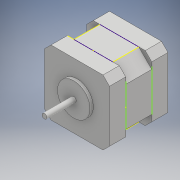
# Autodesk Inventor part: Moteur courroie
Saved by Autodesk Inventor 2018 (Build 220112000, 112)
## iProperties
Created: 2018-04-06
Part Number: Moteur courroie
Material: Générique
Document SubType Name: Modeling
Designer: Dimitri
Density: 1 g/cm^3
Appearance: Par défaut
Author: Dimitri
Autodesk Inventor part; units mm, degrees
ref_plane "YZ Plane" through (0, 0, 0) normal (1, 0, 0) x (0, 1, 0)
ref_plane "XZ Plane" through (0, 0, 0) normal (0, 1, 0) x (-1, 0, 0)
ref_plane "XY Plane" through (0, 0, 0) normal (0, 0, 1) x (1, 0, 0)
sketch "Esquisse1" plane through (0, 0, 0) normal (0, 1, 0) x (-1, 0, 0)
  line L0 (-20, 20) -> (20, 20)
  line L1 (20, 20) -> (20, -20)
  line L2 (20, -20) -> (-20, -20)
  line L3 (-20, -20) -> (-20, 20)
  line L4 (-20, 20) -> (20, -20) construction
  line L5 (20, 20) -> (-20, -20) construction
  point P0 (0, 0)
  dimension "d0" = 40
  dimension "d1" = 40
  constraints: 12 end point, 2 midpoint, 2 parallel, 1 horizontal, 1 perpendicular
  measures "d0" distance of L0.end L1.end
  measures "d1" distance of L1.end L2.end
extrude "Extrusion1" add sketch "Esquisse1" along normal blind 16
chamfer "Chanfrein1" distance 8 angle 45 4 edges at (-20, 8, 20) (20, 8, 20) (20, 8, -20) (-20, 8, -20)
sketch "Esquisse2" plane through (0, 16, 0) normal (0, 1, 0) x (1, 0, 0)
  line L0 (-20, -20) -> (20, -20)
  line L1 (20, -20) -> (20, 20)
  line L2 (20, 20) -> (-20, 20)
  line L3 (-20, 20) -> (-20, -20)
  line L4 (-20, -20) -> (20, 20) construction
  line L5 (20, -20) -> (-20, 20) construction
  point P0 (0, 0)
  dimension "d7" = 40
  constraints: 12 end point, 2 midpoint, 2 parallel, 1 horizontal, 1 perpendicular
  measures "d7" distance of L2.end L1.end
extrude "Extrusion2" add sketch "Esquisse2" along normal blind 10
chamfer "Chanfrein2" distance 4 angle 45 4 edges at (20, 21, -20) (20, 21, 20) (-20, 21, 20) (-20, 21, -20)
sketch "Esquisse3" plane through (0, 0, 0) normal (0, -1, 0) x (1, 0, 0)
  line L0 (20, 20) -> (-20, 20)
  line L1 (-20, 20) -> (-20, -20)
  line L2 (-20, -20) -> (20, -20)
  line L3 (20, -20) -> (20, 20)
  line L4 (20, 20) -> (-20, -20) construction
  line L5 (-20, 20) -> (20, -20) construction
  point P0 (0, 0)
  dimension "d13" = 40
  dimension "d14" = 40
  constraints: 12 end point, 2 midpoint, 2 parallel, 1 horizontal, 1 perpendicular
  measures "d13" distance of L2.end L1.end
  measures "d14" distance of L1.end L0.end
extrude "Extrusion3" add sketch "Esquisse3" along normal blind 10
chamfer "Chanfrein3" distance 4 angle 45 4 edges at (-20, -5, 20) (20, -5, 20) (20, -5, -20) (-20, -5, -20)
sketch "Esquisse4" plane through (0, -10, 0) normal (0, -1, 0) x (1, 0, 0)
  circle A0 centre (0, 0) radius 10
  dimension "d20" = 20
  constraints: 1 centre point, 1 coincident
  measures "d20" diameter of A0
extrude "Extrusion4" add sketch "Esquisse4" along normal blind 2
sketch "Esquisse5" plane through (0, -12, 0) normal (0, -1, 0) x (1, 0, 0)
  circle A0 centre (0, 0) radius 1.5
  dimension "d23" = 3
  constraints: 1 centre point, 1 coincident
  measures "d23" diameter of A0
extrude "Extrusion5" add sketch "Esquisse5" along normal blind 18
sketch "Esquisse6" plane through (12, 16, 20) normal (0, 0, 1) x (1, 0, 0)
  line L0 (0, -16) -> (0, 0) projected
  line L1 (-24, 0) -> (-24, -16) projected
  line L2 (0, 0) -> (-24, 0)
  line L3 (-28, -16) -> (-24, -16) projected
  line L4 (0, -16) -> (-24, -16)
  point P0 (-12, -16)
  constraints: 4 end point, 2 horizontal
sketch "Esquisse7" plane through (20, 16, -12) normal (1, 0, 0) x (0, 0, -1)
  line L0 (0, 0) -> (-25.6172, 0)
  line L1 (0, -16) -> (-25.6172, -16)
  point P0 (-12, -16)
  constraints: 4 end point, 2 horizontal
sketch "Esquisse8" plane through (-12, 16, -20) normal (0, 0, -1) x (-1, 0, 0)
  line L0 (0, 0) -> (0, -16) projected
  line L1 (-24, -16) -> (-24, 0) projected
  line L2 (0, 0) -> (-24, 0)
  line L3 (4, -16) -> (0, -16) projected
  line L4 (0, -16) -> (-24, -16)
  point P0 (-12, -16)
  constraints: 4 end point, 1 collinear, 1 perpendicular
sketch "Esquisse9" plane through (-20, 16, 12) normal (-1, 0, 0) x (0, 0, 1)
  line L0 (0, 0) -> (-24.1988, 0)
  line L1 (0, -16) -> (-24.1988, -16)
  point P0 (-12, -16)
  constraints: 4 end point, 2 horizontal
